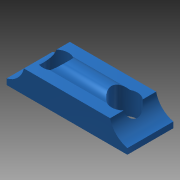
# Autodesk Inventor part: Infill3DLever
Saved by Autodesk Inventor 2015 SP1 (Build 190203100, 203)
## iProperties
Created: 2015-04-28
Part Number: Infill3DLever
Material: Generic
Document SubType Name: Modeling
Designer: Jack
Density: 1 g/cm^3
Appearance: Cyan
Author: Jack
Autodesk Inventor part; units mm, degrees
ref_plane "YZ Plane" through (0, 0, 0) normal (1, 0, 0) x (0, 1, 0)
ref_plane "XZ Plane" through (0, 0, 0) normal (0, 1, 0) x (-1, 0, 0)
sketch "Sketch1" plane through (0, 0, 0) normal (0, 0, 1) x (1, 0, 0)
  line L0 (0, 0) -> (21, 0)
  line L1 (21, 0) -> (21, 8)
  line L2 (21, 8) -> (0, 8)
  line L3 (0, 8) -> (0, 0)
  dimension "d0" = 21
  dimension "d1" = 8
  constraints: 8 end point, 2 horizontal, 2 perpendicular
  measures "d0" distance of L0.start L0.end
  measures "d1" distance of L0.end L1.end
extrude "Extrusion1" add sketch "Sketch1" along normal blind 4
sketch "Sketch2" plane through (0, 8, 0) normal (0, 1, 0) x (1, 0, 0)
  line L0 (0, 0) -> (0, -4) projected
  line L1 (0, -4) -> (21, -4) projected
  arc A0 (3, -4) -> (0, -1) centre (-0.8979, -4.8979) ccw
  line L2 (21, 0) -> (21, -4) projected
  arc A1 (21, -1) -> (18, -4) centre (21.8979, -4.8979) ccw
  dimension "d4" = 4
  dimension "d5" = 1
  dimension "d6" = 3
  dimension "d7" = 3
  constraints: 4 point on circle, 4 point on line, 2 centre point, 1 equal radius, 1 horizontal alignment
  measures "d4" radius of A0
  measures "d5" distance of L0.start A0.end
  measures "d6" distance of L0.end A0.start
  measures "d7" distance of L1.end A1.end
extrude "Extrusion2" cut sketch "Sketch2" against normal up to next
ref_plane "Work Plane2" through (10.5, 0, 0) normal (-1, 0, 0) x (0, 0, 1)
sketch "Sketch5" plane through (10.5, 0, 0) normal (-1, 0, 0) x (0, 0, 1)
  line L0 (4, 8) -> (4, 0) projected
  line L1 (4, 0) -> (4, 8) projected
  arc A0 (4, 2) -> (4, 6) centre (2.5, 4) ccw
  point P0 (0, 0)
  dimension "d25" = 2.5
  dimension "d26" = 1.5
  dimension "d27" = 4
  constraints: 2 point on circle, 2 point on line, 1 centre point
  measures "d25" radius of A0
  measures "d26" distance from line of L0 A0.centre
  measures "d27" vertical distance of L0.start A0.centre
extrude "Extrusion4" add sketch "Sketch5" along normal mid plane 12
sketch "Sketch3" plane through (0, 0, 0) normal (0, 0, -1) x (-1, 0, 0)
  line L0 (-21, 8) -> (0, 8) projected
  line L1 (-21, 0) -> (-21, 8) projected
  point P0 (-4.5, 4)
  point P1 (-16.5, 4)
  dimension "d10" = 12
  dimension "d11" = 4.5
  dimension "d12" = 4
  constraints: 1 horizontal alignment
  measures "d10" distance of point (-4.5, 4) point (-16.5, 4)
  measures "d11" distance from line of L1 point (-16.5, 4)
  measures "d12" distance from line of L0 point (-4.5, 4)
hole "Hole1" at (4.5, 4, 0) at (16.5, 4, 0) direction (0, 0, 1) diameter 4.5 end through all
body "Solid1"
